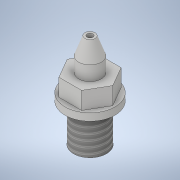
# Autodesk Inventor part: ZKE-Term-Sprung
Saved by Autodesk Inventor 2021 (Build 250183000, 183)
## iProperties
Created: 2020-06-09
Part Number: ZKE-Term-Sprung
Material: Generic
Document SubType Name: Modeling
Designer: lucas
Density: 1 g/cm^3
Appearance: Default
Project: 4Wire-Laser
Author: lucas
Revision Number: ZKE_SPRUNG_19.5mm
Autodesk Inventor part; units mm, degrees
ref_plane "YZ Plane" through (0, 0, 0) normal (1, 0, 0) x (0, 1, 0)
ref_plane "XZ Plane" through (0, 0, 0) normal (0, 1, 0) x (-1, 0, 0)
sketch "Sketch1" plane through (0, 0, 0) normal (0, 1, 0) x (-1, 0, 0)
  circle A0 centre (0, 0) radius 3.9
  dimension "d0" = 7.8
  constraints: 1 centre point
  measures "d0" diameter of A0
extrude "Extrusion1" add sketch "Sketch1" along normal blind 5
ref_plane "Work Plane1" through (0, 11, 0) normal (0, 1, 0) x (1, 0, 0)
sketch "Sketch2" plane through (0, 11, 0) normal (0, 1, 0) x (1, 0, 0)
  circle A0 centre (0, 0) radius 1.75
  dimension "d4" = 3.5
  constraints: 1 centre point
  measures "d4" diameter of A0
loft "Loft1" add profiles "Sketch2" section 1 edges at (3.9, 5, 0)
sketch "Sketch3" plane through (0, 11, 0) normal (0, 1, 0) x (1, 0, 0)
  circle A0 centre (0, 0) radius 1
  dimension "d9" = 2
  constraints: 1 centre point
  measures "d9" diameter of A0
sketch "Sketch4" plane through (0, 0, 0) normal (0, -1, 0) x (1, 0, 0)
  circle A0 centre (0, 0) radius 1.75 projected
  line L0 (7.852, 0) -> (3.926, -6.8)
  line L1 (3.926, -6.8) -> (-3.926, -6.8)
  line L2 (-3.926, -6.8) -> (-7.852, 0)
  line L3 (-7.852, 0) -> (-3.926, 6.8)
  line L4 (-3.926, 6.8) -> (3.926, 6.8)
  line L5 (3.926, 6.8) -> (7.852, 0)
  dimension "d22" = 13.6
  constraints: 12 end point, 1 coincident, 13 other
  measures "d22" distance between parallel lines of L4 L1
extrude "Extrusion2" add sketch "Sketch4" along normal blind 6
sketch "Sketch5" plane through (0, -6, 0) normal (0, -1, 0) x (1, 0, 0)
  circle A0 centre (0, 0) radius 8.6
  dimension "d12" = 17.2
  constraints: 1 centre point
  measures "d12" diameter of A0
extrude "Extrusion3" add sketch "Sketch5" along normal blind 2.5
sketch "Sketch6" plane through (0, -8.5, 0) normal (0, -1, 0) x (1, 0, 0)
  circle A0 centre (0, 0) radius 5.65
  dimension "d15" = 11.3
  constraints: 1 centre point
  measures "d15" diameter of A0
extrude "Extrusion4" add sketch "Sketch6" along normal blind 13
thread "Thread1" size "M14x2" class "6g" standard "ISO Metric profile" full length
extrude "Extrusion5" cut sketch "Sketch3" against normal up to surface (32.5 mm away)
body "Solid1"
